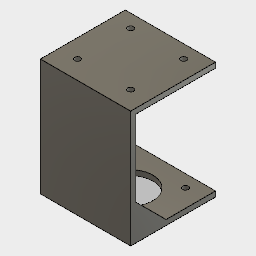
nema-17-mount (Autodesk Fusion 360 design; units mm, degrees)
Autodesk Fusion 360 part; units mm, degrees
sketch "Sketch1" plane through (0, 0, 0) normal (0, 1, 0) x (1, 0, 0)
  line L0 (22.5, 22.5) -> (-22.5, 22.5)
  line L1 (-22.5, 22.5) -> (-22.5, -22.5)
  line L2 (-22.5, -22.5) -> (22.5, -22.5)
  line L3 (22.5, -22.5) -> (22.5, 22.5)
  line L4 (22.5, 22.5) -> (-22.5, -22.5) construction
  line L5 (-22.5, 22.5) -> (22.5, -22.5) construction
  circle A0 centre (0, 0) radius 12.5
  line L6 (15.5, -15.5) -> (-15.5, 15.5) construction
  line L7 (-15.5, -15.5) -> (15.5, 15.5) construction
  circle A1 centre (-15.5, 15.5) radius 1.65
  circle A2 centre (-15.5, -15.5) radius 1.65
  circle A3 centre (15.5, -15.5) radius 1.65
  circle A4 centre (15.5, 15.5) radius 1.65
  dimension "d3" = 45
  dimension "d4" = 45
  dimension "d5" = 25
  dimension "d6" = 31
  dimension "d7" = 31
  dimension "d8" = 3.3
  dimension "d9" = 3.3
  dimension "d10" = 3.3
  dimension "d11" = 3.3
  constraint perpendicular L0 L1
  constraint parallel L0 L2
  constraint parallel L1 L3
  constraint horizontal L0
  constraint coincident L4 A0.centre
  constraint coincident L5 A0.centre
  constraint coincident A0.centre origin
  constraint coincident L6 A0.centre
  constraint coincident L7 A0.centre
  measures "d5" diameter of A0
  measures "d8" diameter of A1
  measures "d9" diameter of A2
  measures "d10" diameter of A3
  measures "d11" diameter of A4
extrude "Extrude1" add sketch "Sketch1" along normal blind 2
sketch "Sketch2" plane through (0, 0, 0) normal (0, 1, 0) x (1, 0, 0)
  line L0 (-22.5, -22.5) -> (22.5, -22.5)
  line L1 (22.5, -22.5) -> (22.5, -25.5)
  line L2 (22.5, -25.5) -> (-22.5, -25.5)
  line L3 (-22.5, -25.5) -> (-22.5, -22.5)
  dimension "d14" = 3
  constraint horizontal L0
  constraint vertical L1
  constraint horizontal L2
  constraint vertical L3
  measures "d14" distance of origin
extrude "Extrude2" add sketch "Sketch2" along normal blind 40
extrude "Extrude3" add 1 faces at (-7.5, 40, 23.5) along direction (0, 1, 0) blind 16
extrude "Extrude4" add 1 faces at (-4.8917, 2, 20.643) along direction (0, 1, 0) blind 1
sketch "Sketch3" plane through (0, 0, 22.5) normal (0, 0, -1) x (-1, 0, 0)
  line L0 (-22.5, 3) -> (22.5, 3)
  line L1 (22.5, 3) -> (22.5, 56)
  line L2 (22.5, 56) -> (-22.5, 56)
  line L3 (-22.5, 56) -> (-22.5, 3)
  line L4 (-22.5, 56) -> (22.5, 56)
  line L5 (22.5, 56) -> (22.5, 53)
  line L6 (22.5, 53) -> (-22.5, 53)
  line L7 (-22.5, 53) -> (-22.5, 56)
  dimension "d21" = 3
  constraint horizontal L4
  constraint vertical L5
  constraint horizontal L6
  constraint vertical L7
  measures "d21" distance of origin
extrude "Extrude5" add sketch "Sketch3" along normal blind 45 contours L1 L2 L3 L4 L5 L6 L7
sketch "Sketch4" plane through (0, 0, 22.5) normal (0, 0, -1) x (-1, 0, 0)
move_face "OffsetFaces1" offset 10 1 faces at (-7.5, 56, 9.5)
move_face "OffsetFaces2" offset -10 1 faces at (-7.5, 53, -7.5)
sketch "Sketch5" plane through (0, 0, 22.5) normal (0, 0, -1) x (-1, 0, 0)
move_body "MoveBody1" bodies 1 to x (1, 0, 0) y (0, 1, 0) z (0, 0, 1) at (0, 0, -50)
sketch "Sketch6" plane through (22.5, 0, 0) normal (1, 0, 0) x (0, 0, -1)
  line L0 (24.5, 0) -> (72.5, 0)
  line L1 (72.5, 0) -> (72.5, 3)
  line L2 (72.5, 3) -> (27.5, 3)
  line L3 (27.5, 3) -> (27.5, 63)
  line L4 (27.5, 63) -> (72.5, 63)
  line L5 (72.5, 63) -> (72.5, 66)
  line L6 (72.5, 66) -> (24.5, 66)
  line L7 (24.5, 66) -> (24.5, 0)
  line L8 (24.5, 0) -> (44.5, 0)
  line L9 (44.5, 0) -> (44.5, 20)
  line L10 (44.5, 20) -> (24.5, 20)
  line L11 (24.5, 20) -> (24.5, 0)
  dimension "d27" = 20
  dimension "d28" = 20
  constraint horizontal L8
  constraint vertical L11
  measures "d27" distance of origin
extrude "Extrude6" add sketch "Sketch6" along normal blind 3
chamfer "Chamfer1" distance 17 angle 45 1 edges at (24, 20, -44.5)
sketch "Sketch7" plane through (-22.5, 0, 0) normal (-1, 0, 0) x (0, 0, 1)
  line L0 (-72.5, 0) -> (-24.5, 0)
  line L1 (-24.5, 0) -> (-24.5, 66)
  line L2 (-24.5, 66) -> (-72.5, 66)
  line L3 (-72.5, 66) -> (-72.5, 63)
  line L4 (-72.5, 63) -> (-27.5, 63)
  line L5 (-27.5, 63) -> (-27.5, 3)
  line L6 (-27.5, 3) -> (-72.5, 3)
  line L7 (-72.5, 3) -> (-72.5, 0)
  line L8 (-24.5, 0) -> (-44.5, 0)
  line L9 (-44.5, 0) -> (-44.5, 20)
  line L10 (-44.5, 20) -> (-24.5, 20)
  line L11 (-24.5, 20) -> (-24.5, 0)
  dimension "d32" = 20
  dimension "d33" = 20
  constraint horizontal L8
  constraint vertical L9
  constraint horizontal L10
  constraint vertical L11
extrude "Extrude7" add sketch "Sketch7" along normal blind 3
chamfer "Chamfer2" distance 17 angle 45 1 edges at (-24, 20, -44.5)
sketch "Sketch8" plane through (0, 66, 0) normal (0, 1, 0) x (-1, 0, 0)
  line L0 (25.5, -24.5) -> (-25.5, -24.5)
  line L1 (-25.5, -24.5) -> (-25.5, -72.5)
  line L2 (-25.5, -72.5) -> (25.5, -72.5)
  line L3 (25.5, -72.5) -> (25.5, -24.5)
  line L4 (-15, -35) -> (15, -65) construction
  line L5 (15, -35) -> (-15, -65) construction
  circle A0 centre (15, -65) radius 1.65
  circle A1 centre (-15, -65) radius 1.65
  circle A2 centre (-15, -35) radius 1.65
  circle A3 centre (15, -35) radius 1.65
  dimension "d37" = 30
  dimension "d38" = 30
  dimension "d39" = 3.3
  dimension "d40" = 3.3
  dimension "d41" = 3.3
  dimension "d42" = 3.3
  constraint coincident L4 origin
  constraint coincident L5 origin
  measures "d39" diameter of A0
  measures "d40" diameter of A1
  measures "d41" diameter of A2
  measures "d42" diameter of A3
extrude "Extrude8" cut sketch "Sketch8" against normal blind 8 contours A0 | A1 | A2 | A3
